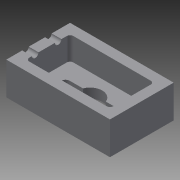
# Autodesk Inventor part: ls-halterung
Saved by Autodesk Inventor 2015 (Build 190159000, 159)
## iProperties
Created: 2014-11-28
Part Number: ls-halterung
Material: Generisch
Document SubType Name: Modeling
Designer: Zephram
Density: 1 g/cm^3
Appearance: Vorgabe
Author: Zephram
Autodesk Inventor part; units mm, degrees
ref_plane "YZ Plane" through (0, 0, 0) normal (1, 0, 0) x (0, 1, 0)
ref_plane "XZ Plane" through (0, 0, 0) normal (0, 1, 0) x (-1, 0, 0)
ref_plane "XY Plane" through (0, 0, 0) normal (0, 0, 1) x (1, 0, 0)
sketch "Skizze1" plane through (0, 0, 0) normal (0, 0, 1) x (1, 0, 0)
  line L0 (0, 22.5879) -> (0, -19.7685)
  line L1 (-28.9042, 0) -> (30.2947, 0)
  line L2 (-15.85, 9.75) -> (15.85, 9.75)
  line L3 (15.85, 9.75) -> (15.85, -9.75)
  line L4 (15.85, -9.75) -> (-15.85, -9.75)
  line L5 (-15.85, -9.75) -> (-15.85, 9.75)
  point P0 (0, 0)
  dimension "d0" = 31.7
  dimension "d1" = 19.5
  constraints: 12 end point, 2 horizontal, 2 parallel, 2 point on line, 1 perpendicular, 1 vertical, 2 other
  measures "d0" distance between parallel lines of L3 L5
  measures "d1" distance between parallel lines of L4 L2
extrude "Extrusion1" add sketch "Skizze1" along normal blind 10
sketch "Skizze2" plane through (0, 0, 10) normal (0, 0, 1) x (1, 0, 0)
  line L0 (-12.85, 6.75) -> (12.85, 6.75)
  line L1 (12.85, 6.75) -> (12.85, -6.75)
  line L2 (12.85, -6.75) -> (-12.85, -6.75)
  line L3 (-12.85, -6.75) -> (-12.85, 6.75)
  line L4 (15.85, -9.75) -> (15.85, 9.75) projected
  line L5 (-15.85, -9.75) -> (15.85, -9.75) projected
  line L6 (-15.85, 9.75) -> (-15.85, -9.75) projected
  line L7 (15.85, 9.75) -> (-15.85, 9.75) projected
  point P0 (0, 0)
  dimension "d4" = 3
  dimension "d5" = 3
  dimension "d6" = 3
  dimension "d7" = 3
  constraints: 8 end point, 2 parallel, 1 horizontal, 1 perpendicular
  measures "d4" distance between parallel lines of L4 L1
  measures "d5" distance between parallel lines of L5 L2
  measures "d6" distance between parallel lines of L6 L3
  measures "d7" distance between parallel lines of L7 L0
extrude "Extrusion2" cut sketch "Skizze2" against normal blind 7 contours L0 L1 L2 L3
sketch "Skizze3" plane through (-15.85, -9.75, 0) normal (-1, 0, 0) x (0, 0, 1)
  line L0 (10, 0) -> (10, 19.5) projected
  arc A0 (10, 13.8534) -> (10, 11.8534) centre (10, 12.8534) ccw
  arc A1 (10, 6.8534) -> (10, 4.8534) centre (10, 5.8534) ccw
  line L1 (10, 19.5) -> (10, 0) projected
  line L2 (-1.0357, 9.3534) -> (13.3763, 9.3534)
  point P0 (0, 9.75)
  dimension "d10" = 7
  dimension "d11" = 1
  dimension "d12" = 1
  constraints: 6 point on line, 4 point on circle, 2 centre point, 2 end point, 1 horizontal, 1 symmetric about line
  measures "d10" distance of A1.centre A0.centre
  measures "d11" radius of A0
  measures "d12" radius of A1
extrude "Extrusion3" cut sketch "Skizze3" against normal blind 7
fillet "Rundung1" radius 1 4 edges at (12.85, -6.75, 6.5) (12.85, 6.75, 6.5) (-12.85, 6.75, 6.5) (-12.85, -6.75, 6.5)
sketch "Skizze4" plane through (0, 0, 3) normal (0, 0, 1) x (1, 0, 0)
  arc A0 (12.85, 5.75) -> (11.85, 6.75) centre (11.85, 5.75) ccw projected
  line L0 (11.85, 6.75) -> (-11.85, 6.75) projected
  arc A1 (-11.85, 6.75) -> (-12.85, 5.75) centre (-11.85, 5.75) ccw projected
  line L1 (-12.85, 5.75) -> (-12.85, -5.75) projected
  arc A2 (-12.85, -5.75) -> (-11.85, -6.75) centre (-11.85, -5.75) ccw projected
  line L2 (-11.85, -6.75) -> (11.85, -6.75) projected
  arc A3 (11.85, -6.75) -> (12.85, -5.75) centre (11.85, -5.75) ccw projected
  line L3 (12.85, -5.75) -> (12.85, 5.75) projected
  line L4 (15.85, 9.75) -> (15.85, -9.75) projected
  line L5 (15.85, -9.75) -> (-15.85, -9.75) projected
  line L6 (-15.85, -9.75) -> (-15.85, 9.75) projected
  line L7 (-15.85, 9.75) -> (15.85, 9.75) projected
  circle A4 centre (-7.5, 0) radius 2.5
  circle A5 centre (7.5, 0) radius 2.5
  circle A6 centre (-7.5, 0) radius 1.35
  circle A7 centre (7.5, 0) radius 1.35
  circle A8 centre (0, 0) radius 3.75
  circle A9 centre (0, 0) radius 1.35
  line L8 (-7.5, 1.35) -> (0, 1.35)
  line L9 (-7.5, -1.35) -> (0, -1.35)
  line L10 (0, 1.35) -> (7.5, 1.35)
  line L11 (7.5, -1.35) -> (0, -1.35)
  dimension "d16" = 7.5
  dimension "d17" = 7.5
  dimension "d18" = 5
  dimension "d19" = 5
  dimension "d20" = 2.7
  dimension "d21" = 2.7
  dimension "d22" = 7.5
  dimension "d23" = 2.7
  constraints: 8 end point, 6 centre point, 6 coincident, 6 point on circle, 4 tangent, 1 parallel, 1 point on line
  measures "d16" distance of point (7.5, 0) point (0, 0)
  measures "d17" distance of point (-7.5, 0) point (0, 0)
  measures "d18" diameter of A4
  measures "d19" diameter of A5
  measures "d20" diameter of A6
  measures "d21" diameter of A7
  measures "d22" diameter of A8
  measures "d23" diameter of A9
extrude "Extrusion4" cut sketch "Skizze4" against normal blind 5 contours A4 L9 A6 L8 | A4 L8 A8 L9 | A6 | L8 A9 L9 A8 | A8 L10 L8 | L9 L11 A8 | L10 A5 L11 A8 | A8 L11 A9 L10 | A9 | L10 A7 L11 A5 | A7 picked at (-5.3984, -0.1575) picked at (5.3974, -0.0542)
